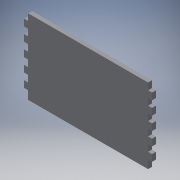
# Autodesk Inventor part: полуверх 2
Saved by Autodesk Inventor 2019 (Build 230136000, 136)
## iProperties
Created: 2022-02-24
Part Number: полуверх 2
Material: Типовые
Document SubType Name: Modeling
Designer: korsh
Density: 1 g/cm^3
Appearance: По умолчанию
Author: korsh
Autodesk Inventor part; units mm, degrees
ref_plane "YZ Plane" through (0, 0, 0) normal (1, 0, 0) x (0, 1, 0)
ref_plane "XZ Plane" through (0, 0, 0) normal (0, 1, 0) x (-1, 0, 0)
ref_plane "XY Plane" through (0, 0, 0) normal (0, 0, 1) x (1, 0, 0)
ref_plane "РабПлоскость1" through (0, -60, 0) normal (0, 0, 1) x (1, 0, 0)
sketch "Эскиз1" plane through (0, -60, 0) normal (0, 0, 1) x (1, 0, 0)
  line L0 (186, 0) -> (186, 10) projected
  line L1 (186, 0) -> (186, 10) projected
  line L2 (186, 0) -> (192, 0) projected
  line L3 (192, 10) -> (192, 0) projected
  line L4 (186, 10) -> (192, 10) projected
  line L5 (186, 20) -> (186, 30) projected
  line L6 (186, 20) -> (192, 20) projected
  line L7 (192, 30) -> (192, 20) projected
  line L8 (186, 30) -> (192, 30) projected
  line L9 (186, 40) -> (186, 50) projected
  line L10 (186, 40) -> (192, 40) projected
  line L11 (192, 50) -> (192, 40) projected
  line L12 (186, 50) -> (192, 50) projected
  line L13 (186, 60) -> (186, 70) projected
  line L14 (186, 60) -> (192, 60) projected
  line L15 (192, 70) -> (192, 60) projected
  line L16 (186, 70) -> (192, 70) projected
  line L17 (186, 80) -> (186, 90) projected
  line L18 (186, 80) -> (192, 80) projected
  line L19 (192, 90) -> (192, 80) projected
  line L20 (186, 90) -> (192, 90) projected
  line L21 (186, 90) -> (186, 100) projected
  line L22 (186, -12.5234) -> (186, 0) projected
  line L23 (6, 0) -> (6, -12.5234) projected
  line L24 (0, 0) -> (0, 10) projected
  line L25 (0, 0) -> (6, 0) projected
  line L26 (6, 10) -> (6, 0) projected
  line L27 (0, 10) -> (6, 10) projected
  line L28 (0, 20) -> (0, 30) projected
  line L29 (0, 20) -> (6, 20) projected
  line L30 (6, 30) -> (6, 20) projected
  line L31 (0, 30) -> (6, 30) projected
  line L32 (0, 60) -> (0, 70) projected
  line L33 (0, 60) -> (6, 60) projected
  line L34 (6, 70) -> (6, 60) projected
  line L35 (0, 70) -> (6, 70) projected
  line L36 (0, 80) -> (0, 90) projected
  line L37 (0, 80) -> (6, 80) projected
  line L38 (6, 90) -> (6, 80) projected
  line L39 (0, 90) -> (6, 90) projected
  line L40 (6, 100) -> (6, 90) projected
  line L41 (0, 40) -> (0, 50) projected
  line L42 (0, 40) -> (6, 40) projected
  line L43 (6, 50) -> (6, 40) projected
  line L44 (0, 50) -> (6, 50) projected
  line L45 (186, -12.5234) -> (6, -12.5234)
  line L46 (6, -12.5234) -> (6, 100)
  line L47 (6, 100) -> (186, 100)
  line L48 (186, 100) -> (186, -12.5234)
  constraints: 8 end point, 2 parallel, 1 horizontal, 1 perpendicular
extrude "Выдавливание1" add sketch "Эскиз1" along normal blind 6
